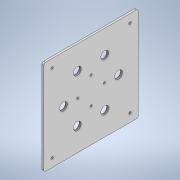
# Autodesk Inventor part: Plate
Saved by Autodesk Inventor 2022 (Build 260153000, 153)
## iProperties
Created: 2022-03-14
Part Number: Plate
Material: Generic
Document SubType Name: Modeling
Designer: ultra
Density: 1 g/cm^3
Appearance: Default
Author: ultra
Autodesk Inventor part; units mm, degrees
ref_plane "YZ Plane" through (0, 0, 0) normal (1, 0, 0) x (0, 1, 0)
ref_plane "XZ Plane" through (0, 0, 0) normal (0, 1, 0) x (-1, 0, 0)
ref_plane "XY Plane" through (0, 0, 0) normal (0, 0, 1) x (1, 0, 0)
sketch "Sketch1" plane through (0, 0, 0) normal (1, 0, 0) x (0, 1, 0)
  line L0 (-76.2, 76.2) -> (76.2, 76.2)
  line L1 (76.2, 76.2) -> (76.2, -76.2)
  line L2 (76.2, -76.2) -> (-76.2, -76.2)
  line L3 (-76.2, -76.2) -> (-76.2, 76.2)
  circle A0 centre (62.8611, 62.86) radius 2.032
  circle A1 centre (-62.8625, -62.8636) radius 2.032
  circle A2 centre (-0.0007, -88.9018) radius 2.032
  circle A3 centre (-62.8625, 62.86) radius 2.032
  circle A4 centre (88.8993, -0.0018) radius 2.032
  circle A5 centre (-88.9007, -0.0018) radius 2.032
  circle A6 centre (62.8611, -62.8636) radius 2.032
  circle A7 centre (-0.0007, 88.8982) radius 2.032
  circle A8 centre (-0.0007, -0.0018) radius 6.35
  dimension "d0" = 152.4
  dimension "d1" = 152.4
  dimension "d5" = 12.7
  constraints: 9 centre point, 8 end point, 2 parallel, 1 horizontal, 1 perpendicular
  measures "d0" distance of L1.end L2.end
  measures "d1" distance of L0.end L1.end
  measures "d5" diameter of A8
extrude "Extrusion2" add sketch "Sketch1" along normal blind 3.175 contours L0 L1 L2 L3 | A8
fillet "Fillet2" radius 3.175 4 edges at (1.5875, 76.2, 76.2) (1.5875, 76.2, -76.2) (1.5875, -76.2, 76.2) (1.5875, -76.2, -76.2)
sketch "Sketch2" plane through (3.175, 0, 0) normal (1, 0, 0) x (0, 0, -1)
  line L0 (-50.8, -50.8) -> (50.8, -50.8)
  line L1 (50.8, -50.8) -> (50.8, 50.8)
  line L2 (50.8, 50.8) -> (-50.8, 50.8)
  line L3 (-50.8, 50.8) -> (-50.8, -50.8)
  line L4 (-50.8, -50.8) -> (50.8, 50.8) construction
  line L5 (50.8, -50.8) -> (-50.8, 50.8) construction
  circle A0 centre (0, 0) radius 12.7
  line L6 (-12.7, 0) -> (-50.8, 38.1)
  line L7 (0, 12.7) -> (-38.1, 50.8)
  line L8 (-38.1, 50.8) -> (0, 12.7)
  line L9 (38.1, 50.8) -> (0, 12.7)
  line L10 (12.7, 0) -> (50.8, 38.1)
  line L11 (12.7, 0) -> (50.8, -38.1)
  line L12 (0, -12.7) -> (38.1, -50.8)
  line L13 (0, -12.7) -> (-38.1, -50.8)
  line L14 (-12.7, 0) -> (-50.8, -38.1)
  dimension "d9" = 101.6
  dimension "d10" = 101.6
  dimension "d11" = 25.4
  constraints: 30 end point, 10 point on line, 5 parallel, 4 point on circle, 2 midpoint, 2 perpendicular, 1 centre point, 1 coincident, 1 collinear, 1 horizontal
  measures "d9" distance of L2.end L1.end
  measures "d10" distance of L1.end L0.end
  measures "d11" diameter of A0
extrude "Extrusion3" [suppressed]
fillet "Fillet3" [suppressed]
sketch "Sketch3" plane through (3.175, 0, 0) normal (1, 0, 0) x (0, 0, -1)
  circle A0 centre (-22.225, -38.4948) radius 6.35
  circle A1 centre (-44.45, 0) radius 6.35
  circle A2 centre (22.225, -38.4948) radius 6.35
  circle A3 centre (-22.225, 38.4948) radius 6.35
  circle A4 centre (22.225, 38.4948) radius 6.35
  circle A5 centre (44.45, 0) radius 6.35
  point P0 (0, 0)
  constraints: 6 centre point
extrude "Extrusion4" cut sketch "Sketch3" against normal blind 25.4
sketch "Sketch4" plane through (3.175, 0, 0) normal (1, 0, 0) x (0, 0, -1)
  arc A0 (23.2155, 2.1696) -> (22.9916, -2.3228) centre (21.5668, 0) ccw
  line L0 (23.2155, 2.1696) -> (2.1696, 23.2155)
  arc A1 (-2.3228, 22.9916) -> (2.1696, 23.2155) centre (0, 21.5668) ccw
  line L1 (-2.3228, 22.9916) -> (-22.9916, 2.3228)
  arc A2 (-21.0224, -2.6701) -> (-22.9916, 2.3228) centre (-21.5668, 0) ccw
  arc A3 (-21.0026, -2.6855) -> (-21.0224, -2.6701) centre (-21.0733, -2.7562) ccw
  line L2 (-21.0026, -2.6855) -> (-2.6855, -21.0026)
  arc A4 (-2.6701, -21.0224) -> (-2.6855, -21.0026) centre (-2.7562, -21.0733) ccw
  arc A5 (2.3228, -22.9916) -> (-2.6701, -21.0224) centre (0, -21.5668) ccw
  line L3 (2.3228, -22.9916) -> (22.9916, -2.3228)
  circle A6 centre (3.0052, -18.703) radius 0.6
  circle A7 centre (4.1012, -19.799) radius 0.6
  circle A8 centre (6.8364, 2.2749) radius 0.5
  line L4 (-6.1377, 16.2493) -> (-7.0852, 17.1968)
  arc A9 (-6.1377, 16.1362) -> (-6.1377, 16.2493) centre (-6.1943, 16.1927) ccw
  line L5 (-7.0852, 15.1887) -> (-6.1377, 16.1362)
  arc A10 (-7.1983, 15.1887) -> (-7.0852, 15.1887) centre (-7.1418, 15.2452) ccw
  line L6 (-8.1459, 16.1362) -> (-7.1983, 15.1887)
  arc A11 (-8.1459, 16.2493) -> (-8.1459, 16.1362) centre (-8.0893, 16.1927) ccw
  line L7 (-7.1983, 17.1968) -> (-8.1459, 16.2493)
  arc A12 (-7.0852, 17.1968) -> (-7.1983, 17.1968) centre (-7.1418, 17.1403) ccw
  line L8 (8.8176, 15.6483) -> (7.8701, 16.5958)
  arc A13 (8.8176, 15.5351) -> (8.8176, 15.6483) centre (8.7611, 15.5917) ccw
  line L9 (7.8701, 14.5876) -> (8.8176, 15.5351)
  arc A14 (7.757, 14.5876) -> (7.8701, 14.5876) centre (7.8135, 14.6442) ccw
  line L10 (6.8094, 15.5351) -> (7.757, 14.5876)
  arc A15 (6.8094, 15.6483) -> (6.8094, 15.5351) centre (6.866, 15.5917) ccw
  line L11 (7.757, 16.5958) -> (6.8094, 15.6483)
  arc A16 (7.8701, 16.5958) -> (7.757, 16.5958) centre (7.8135, 16.5392) ccw
  line L12 (19.601, 4.7235) -> (18.6535, 5.671)
  arc A17 (19.601, 4.6103) -> (19.601, 4.7235) centre (19.5444, 4.6669) ccw
  line L13 (18.6535, 3.6628) -> (19.601, 4.6103)
  arc A18 (18.5403, 3.6628) -> (18.6535, 3.6628) centre (18.5969, 3.7194) ccw
  line L14 (17.5928, 4.6103) -> (18.5403, 3.6628)
  arc A19 (17.5928, 4.7235) -> (17.5928, 4.6103) centre (17.6494, 4.6669) ccw
  line L15 (18.5403, 5.671) -> (17.5928, 4.7235)
  arc A20 (18.6535, 5.671) -> (18.5403, 5.671) centre (18.5969, 5.6144) ccw
  line L16 (15.8533, 4.5821) -> (14.9058, 5.5296)
  arc A21 (15.8533, 4.4689) -> (15.8533, 4.5821) centre (15.7968, 4.5255) ccw
  line L17 (14.9058, 3.5214) -> (15.8533, 4.4689)
  arc A22 (14.7927, 3.5214) -> (14.9058, 3.5214) centre (14.8492, 3.578) ccw
  line L18 (13.8452, 4.4689) -> (14.7927, 3.5214)
  arc A23 (13.8452, 4.5821) -> (13.8452, 4.4689) centre (13.9017, 4.5255) ccw
  line L19 (14.7927, 5.5296) -> (13.8452, 4.5821)
  arc A24 (14.9058, 5.5296) -> (14.7927, 5.5296) centre (14.8492, 5.473) ccw
  line L20 (16.419, 0.1273) -> (15.4715, 1.0748)
  arc A25 (16.419, 0.0141) -> (16.419, 0.1273) centre (16.3625, 0.0707) ccw
  line L21 (15.4715, -0.9334) -> (16.419, 0.0141)
  arc A26 (15.3584, -0.9334) -> (15.4715, -0.9334) centre (15.4149, -0.8768) ccw
  line L22 (14.4108, 0.0141) -> (15.3584, -0.9334)
  arc A27 (14.4108, 0.1273) -> (14.4108, 0.0141) centre (14.4674, 0.0707) ccw
  line L23 (15.3584, 1.0748) -> (14.4108, 0.1273)
  arc A28 (15.4715, 1.0748) -> (15.3584, 1.0748) centre (15.4149, 1.0182) ccw
  circle A29 centre (16.122, -7.2832) radius 0.75
  circle A30 centre (-6.5407, -11.7733) radius 0.6
  circle A31 centre (-7.6014, -10.7127) radius 0.6
  circle A32 centre (-8.6621, -9.652) radius 0.6
  circle A33 centre (-8.8035, -12.4097) radius 0.5
  line L24 (18.9292, -5.4235) -> (17.9817, -4.476)
  arc A34 (18.9292, -5.5366) -> (18.9292, -5.4235) centre (18.8727, -5.4801) ccw
  line L25 (17.9817, -6.4842) -> (18.9292, -5.5366)
  arc A35 (17.8686, -6.4842) -> (17.9817, -6.4842) centre (17.9252, -6.4276) ccw
  line L26 (16.9211, -5.5366) -> (17.8686, -6.4842)
  arc A36 (16.9211, -5.4235) -> (16.9211, -5.5366) centre (16.9776, -5.4801) ccw
  line L27 (17.8686, -4.476) -> (16.9211, -5.4235)
  arc A37 (17.9817, -4.476) -> (17.8686, -4.476) centre (17.9252, -4.5326) ccw
  line L28 (-4.2144, 14.326) -> (-5.1619, 15.2735)
  arc A38 (-4.2144, 14.2128) -> (-4.2144, 14.326) centre (-4.2709, 14.2694) ccw
  line L29 (-5.1619, 13.2653) -> (-4.2144, 14.2128)
  arc A39 (-5.275, 13.2653) -> (-5.1619, 13.2653) centre (-5.2184, 13.3219) ccw
  line L30 (-6.2225, 14.2128) -> (-5.275, 13.2653)
  arc A40 (-6.2225, 14.326) -> (-6.2225, 14.2128) centre (-6.166, 14.2694) ccw
  line L31 (-5.275, 15.2735) -> (-6.2225, 14.326)
  arc A41 (-5.1619, 15.2735) -> (-5.275, 15.2735) centre (-5.2184, 15.2169) ccw
  line L32 (7.3618, 0.623) -> (8.3055, 1.5667)
  arc A42 (7.2487, 0.623) -> (7.3618, 0.623) centre (7.3053, 0.6795) ccw
  line L33 (6.8654, 1.0063) -> (7.2487, 0.623)
  arc A43 (6.8654, 1.1194) -> (6.8654, 1.0063) centre (6.922, 1.0629) ccw
  line L34 (7.8091, 2.0631) -> (6.8654, 1.1194)
  arc A44 (7.9222, 2.0631) -> (7.8091, 2.0631) centre (7.8657, 2.0066) ccw
  line L35 (8.3055, 1.6798) -> (7.9222, 2.0631)
  arc A45 (8.3055, 1.5667) -> (8.3055, 1.6798) centre (8.249, 1.6232) ccw
  line L36 (12.9068, -4.7667) -> (14.116, -3.5576)
  arc A46 (12.7937, -4.7667) -> (12.9068, -4.7667) centre (12.8503, -4.7101) ccw
  line L37 (12.0957, -4.0687) -> (12.7937, -4.7667)
  arc A47 (12.0957, -3.9555) -> (12.0957, -4.0687) centre (12.1522, -4.0121) ccw
  line L38 (13.3048, -2.7464) -> (12.0957, -3.9555)
  arc A48 (13.4179, -2.7464) -> (13.3048, -2.7464) centre (13.3614, -2.803) ccw
  line L39 (14.116, -3.4444) -> (13.4179, -2.7464)
  arc A49 (14.116, -3.5576) -> (14.116, -3.4444) centre (14.0594, -3.501) ccw
  line L40 (6.6373, -11.9558) -> (4.8803, -13.7127)
  arc A50 (6.8494, -11.9558) -> (6.6373, -11.9558) centre (6.7433, -12.0618) ccw
  line L41 (7.3, -12.4064) -> (6.8494, -11.9558)
  arc A51 (7.3, -12.6185) -> (7.3, -12.4064) centre (7.194, -12.5125) ccw
  line L42 (5.5431, -14.3755) -> (7.3, -12.6185)
  arc A52 (5.3309, -14.3755) -> (5.5431, -14.3755) centre (5.437, -14.2694) ccw
  line L43 (4.8803, -13.9248) -> (5.3309, -14.3755)
  arc A53 (4.8803, -13.7127) -> (4.8803, -13.9248) centre (4.9864, -13.8188) ccw
  line L44 (-10.9165, -1.3583) -> (-10.3201, -0.7619)
  arc A54 (-11.0296, -1.3583) -> (-10.9165, -1.3583) centre (-10.973, -1.3017) ccw
  line L45 (-11.2566, -1.1313) -> (-11.0296, -1.3583)
  arc A55 (-11.2566, -1.0181) -> (-11.2566, -1.1313) centre (-11.2001, -1.0747) ccw
  line L46 (-10.6602, -0.4217) -> (-11.2566, -1.0181)
  arc A56 (-10.5471, -0.4217) -> (-10.6602, -0.4217) centre (-10.6037, -0.4783) ccw
  line L47 (-10.3201, -0.6487) -> (-10.5471, -0.4217)
  arc A57 (-10.3201, -0.7619) -> (-10.3201, -0.6487) centre (-10.3766, -0.7053) ccw
  line L48 (-10.4537, -1.8887) -> (-10.2266, -2.1157)
  arc A58 (-10.4537, -1.7755) -> (-10.4537, -1.8887) centre (-10.3971, -1.8321) ccw
  line L49 (-9.8573, -1.1791) -> (-10.4537, -1.7755)
  arc A59 (-9.7441, -1.1791) -> (-9.8573, -1.1791) centre (-9.8007, -1.2357) ccw
  line L50 (-9.5171, -1.4061) -> (-9.7441, -1.1791)
  arc A60 (-9.5171, -1.5193) -> (-9.5171, -1.4061) centre (-9.5737, -1.4627) ccw
  line L51 (-10.1135, -2.1157) -> (-9.5171, -1.5193)
  arc A61 (-10.2266, -2.1157) -> (-10.1135, -2.1157) centre (-10.1701, -2.0591) ccw
  line L52 (-4.4405, 1.0113) -> (-4.2546, 0.8254)
  arc A62 (-4.4405, 1.1244) -> (-4.4405, 1.0113) centre (-4.384, 1.0679) ccw
  line L53 (-3.9397, 1.6252) -> (-4.4405, 1.1244)
  arc A63 (-3.8266, 1.6252) -> (-3.9397, 1.6252) centre (-3.8832, 1.5686) ccw
  line L54 (-3.6407, 1.4393) -> (-3.8266, 1.6252)
  arc A64 (-3.6407, 1.3261) -> (-3.6407, 1.4393) centre (-3.6972, 1.3827) ccw
  line L55 (-4.1415, 0.8254) -> (-3.6407, 1.3261)
  arc A65 (-4.2546, 0.8254) -> (-4.1415, 0.8254) centre (-4.198, 0.8819) ccw
  line L56 (-8.9918, 6.0077) -> (-8.8058, 5.8218)
  arc A66 (-8.9918, 6.1208) -> (-8.9918, 6.0077) centre (-8.9352, 6.0642) ccw
  line L57 (-8.491, 6.6216) -> (-8.9918, 6.1208)
  arc A67 (-8.3778, 6.6216) -> (-8.491, 6.6216) centre (-8.4344, 6.565) ccw
  line L58 (-8.1919, 6.4357) -> (-8.3778, 6.6216)
  arc A68 (-8.1919, 6.3225) -> (-8.1919, 6.4357) centre (-8.2485, 6.3791) ccw
  line L59 (-8.6927, 5.8218) -> (-8.1919, 6.3225)
  arc A69 (-8.8058, 5.8218) -> (-8.6927, 5.8218) centre (-8.7493, 5.8783) ccw
  line L60 (2.8669, 3.1449) -> (3.0528, 2.9589)
  arc A70 (2.8669, 3.258) -> (2.8669, 3.1449) centre (2.9235, 3.2014) ccw
  line L61 (3.3677, 3.7588) -> (2.8669, 3.258)
  arc A71 (3.4808, 3.7588) -> (3.3677, 3.7588) centre (3.4243, 3.7022) ccw
  line L62 (3.6668, 3.5729) -> (3.4808, 3.7588)
  arc A72 (3.6668, 3.4597) -> (3.6668, 3.5729) centre (3.6102, 3.5163) ccw
  line L63 (3.166, 2.9589) -> (3.6668, 3.4597)
  arc A73 (3.0528, 2.9589) -> (3.166, 2.9589) centre (3.1094, 3.0155) ccw
  line L64 (4.4253, 1.5865) -> (4.6112, 1.4005)
  arc A74 (4.4253, 1.6996) -> (4.4253, 1.5865) centre (4.4819, 1.643) ccw
  line L65 (4.9261, 2.2004) -> (4.4253, 1.6996)
  arc A75 (5.0392, 2.2004) -> (4.9261, 2.2004) centre (4.9827, 2.1438) ccw
  line L66 (5.2252, 2.0145) -> (5.0392, 2.2004)
  arc A76 (5.2252, 1.9013) -> (5.2252, 2.0145) centre (5.1686, 1.9579) ccw
  line L67 (4.7244, 1.4005) -> (5.2252, 1.9013)
  arc A77 (4.6112, 1.4005) -> (4.7244, 1.4005) centre (4.6678, 1.4571) ccw
  line L68 (7.7498, 0.1218) -> (7.9358, -0.0641)
  arc A78 (7.7498, 0.235) -> (7.7498, 0.1218) centre (7.8064, 0.1784) ccw
  line L69 (8.2506, 0.7358) -> (7.7498, 0.235)
  arc A79 (8.3638, 0.7358) -> (8.2506, 0.7358) centre (8.3072, 0.6792) ccw
  line L70 (8.5497, 0.5498) -> (8.3638, 0.7358)
  arc A80 (8.5497, 0.4367) -> (8.5497, 0.5498) centre (8.4931, 0.4933) ccw
  line L71 (8.0489, -0.0641) -> (8.5497, 0.4367)
  arc A81 (7.9358, -0.0641) -> (8.0489, -0.0641) centre (7.9923, -0.0075) ccw
  line L72 (11.3694, -3.4478) -> (11.5553, -3.6337)
  arc A82 (11.3694, -3.3347) -> (11.3694, -3.4478) centre (11.426, -3.3912) ccw
  line L73 (11.8702, -2.8339) -> (11.3694, -3.3347)
  arc A83 (11.9833, -2.8339) -> (11.8702, -2.8339) centre (11.9268, -2.8904) ccw
  line L74 (12.1692, -3.0198) -> (11.9833, -2.8339)
  arc A84 (12.1692, -3.1329) -> (12.1692, -3.0198) centre (12.1127, -3.0764) ccw
  line L75 (11.6685, -3.6337) -> (12.1692, -3.1329)
  arc A85 (11.5553, -3.6337) -> (11.6685, -3.6337) centre (11.6119, -3.5771) ccw
  line L76 (7.2531, -10.8075) -> (7.439, -10.9935)
  arc A86 (7.2531, -10.6944) -> (7.2531, -10.8075) centre (7.3097, -10.751) ccw
  line L77 (7.7539, -10.1936) -> (7.2531, -10.6944)
  arc A87 (7.867, -10.1936) -> (7.7539, -10.1936) centre (7.8105, -10.2502) ccw
  line L78 (8.053, -10.3795) -> (7.867, -10.1936)
  arc A88 (8.053, -10.4927) -> (8.053, -10.3795) centre (7.9964, -10.4361) ccw
  line L79 (7.5522, -10.9935) -> (8.053, -10.4927)
  arc A89 (7.439, -10.9935) -> (7.5522, -10.9935) centre (7.4956, -10.9369) ccw
  line L80 (8.0117, -11.5935) -> (8.2265, -11.8083)
  arc A90 (8.0117, -11.4804) -> (8.0117, -11.5935) centre (8.0683, -11.537) ccw
  line L81 (8.5536, -10.9385) -> (8.0117, -11.4804)
  arc A91 (8.6668, -10.9385) -> (8.5536, -10.9385) centre (8.6102, -10.995) ccw
  line L82 (8.8816, -11.1533) -> (8.6668, -10.9385)
  arc A92 (8.8816, -11.2664) -> (8.8816, -11.1533) centre (8.825, -11.2098) ccw
  line L83 (8.3396, -11.8083) -> (8.8816, -11.2664)
  arc A93 (8.2265, -11.8083) -> (8.3396, -11.8083) centre (8.2831, -11.7518) ccw
  line L84 (-8.0565, 2.0509) -> (-7.8655, 2.2419)
  arc A94 (-8.1696, 2.0509) -> (-8.0565, 2.0509) centre (-8.1131, 2.1075) ccw
  line L85 (-8.6663, 2.5475) -> (-8.1696, 2.0509)
  arc A95 (-8.6663, 2.6607) -> (-8.6663, 2.5475) centre (-8.6097, 2.6041) ccw
  line L86 (-8.4753, 2.8517) -> (-8.6663, 2.6607)
  arc A96 (-8.3622, 2.8517) -> (-8.4753, 2.8517) centre (-8.4187, 2.7951) ccw
  line L87 (-7.8655, 2.355) -> (-8.3622, 2.8517)
  arc A97 (-7.8655, 2.2419) -> (-7.8655, 2.355) centre (-7.9221, 2.2985) ccw
  line L88 (-6.485, 0.2962) -> (-5.9884, -0.2005)
  arc A98 (-6.485, 0.4093) -> (-6.485, 0.2962) centre (-6.4285, 0.3527) ccw
  line L89 (-6.294, 0.6003) -> (-6.485, 0.4093)
  arc A99 (-6.1809, 0.6003) -> (-6.294, 0.6003) centre (-6.2375, 0.5437) ccw
  line L90 (-5.6842, 0.1036) -> (-6.1809, 0.6003)
  arc A100 (-5.6842, -0.0095) -> (-5.6842, 0.1036) centre (-5.7408, 0.0471) ccw
  line L91 (-5.8752, -0.2005) -> (-5.6842, -0.0095)
  arc A101 (-5.9884, -0.2005) -> (-5.8752, -0.2005) centre (-5.9318, -0.1439) ccw
  line L92 (-8.0538, -3.0609) -> (-7.5571, -3.5576)
  arc A102 (-8.0538, -2.9478) -> (-8.0538, -3.0609) centre (-7.9972, -3.0044) ccw
  line L93 (-7.8627, -2.7568) -> (-8.0538, -2.9478)
  arc A103 (-7.7496, -2.7568) -> (-7.8627, -2.7568) centre (-7.8062, -2.8133) ccw
  line L94 (-7.253, -3.2534) -> (-7.7496, -2.7568)
  arc A104 (-7.253, -3.3666) -> (-7.253, -3.2534) centre (-7.3095, -3.31) ccw
  line L95 (-7.444, -3.5576) -> (-7.253, -3.3666)
  arc A105 (-7.5571, -3.5576) -> (-7.444, -3.5576) centre (-7.5005, -3.501) ccw
  line L96 (10.6894, 0.9692) -> (11.186, 0.4725)
  arc A106 (10.6894, 1.0823) -> (10.6894, 0.9692) centre (10.746, 1.0257) ccw
  line L97 (10.8804, 1.2733) -> (10.6894, 1.0823)
  arc A107 (10.9935, 1.2733) -> (10.8804, 1.2733) centre (10.937, 1.2167) ccw
  line L98 (11.4902, 0.7766) -> (10.9935, 1.2733)
  arc A108 (11.4902, 0.6635) -> (11.4902, 0.7766) centre (11.4336, 0.7201) ccw
  line L99 (11.2992, 0.4725) -> (11.4902, 0.6635)
  arc A109 (11.186, 0.4725) -> (11.2992, 0.4725) centre (11.2426, 0.5291) ccw
  line L100 (7.9785, -2.1827) -> (8.4752, -2.6794)
  arc A110 (7.9785, -2.0696) -> (7.9785, -2.1827) centre (8.0351, -2.1261) ccw
  line L101 (8.1696, -1.8785) -> (7.9785, -2.0696)
  arc A111 (8.2827, -1.8785) -> (8.1696, -1.8785) centre (8.2261, -1.9351) ccw
  line L102 (8.7793, -2.3752) -> (8.2827, -1.8785)
  arc A112 (8.7793, -2.4883) -> (8.7793, -2.3752) centre (8.7228, -2.4318) ccw
  line L103 (8.5883, -2.6794) -> (8.7793, -2.4883)
  arc A113 (8.4752, -2.6794) -> (8.5883, -2.6794) centre (8.5318, -2.6228) ccw
  line L104 (10.502, -8.0563) -> (10.9987, -8.5529)
  arc A114 (10.502, -7.9431) -> (10.502, -8.0563) centre (10.5586, -7.9997) ccw
  line L105 (10.693, -7.7521) -> (10.502, -7.9431)
  arc A115 (10.8061, -7.7521) -> (10.693, -7.7521) centre (10.7496, -7.8087) ccw
  line L106 (11.3028, -8.2488) -> (10.8061, -7.7521)
  arc A116 (11.3028, -8.3619) -> (11.3028, -8.2488) centre (11.2462, -8.3054) ccw
  line L107 (11.1118, -8.5529) -> (11.3028, -8.3619)
  arc A117 (10.9987, -8.5529) -> (11.1118, -8.5529) centre (11.0552, -8.4964) ccw
  line L108 (9.7298, -8.8285) -> (10.2265, -9.3251)
  arc A118 (9.7298, -8.7153) -> (9.7298, -8.8285) centre (9.7864, -8.7719) ccw
  line L109 (9.9208, -8.5243) -> (9.7298, -8.7153)
  arc A119 (10.034, -8.5243) -> (9.9208, -8.5243) centre (9.9774, -8.5809) ccw
  line L110 (10.5306, -9.021) -> (10.034, -8.5243)
  arc A120 (10.5306, -9.1341) -> (10.5306, -9.021) centre (10.474, -9.0776) ccw
  line L111 (10.3396, -9.3251) -> (10.5306, -9.1341)
  arc A121 (10.2265, -9.3251) -> (10.3396, -9.3251) centre (10.283, -9.2686) ccw
  line L112 (8.8271, -9.6036) -> (9.4328, -10.2093)
  arc A122 (8.8271, -9.4905) -> (8.8271, -9.6036) centre (8.8837, -9.5471) ccw
  line L113 (9.1377, -9.1799) -> (8.8271, -9.4905)
  arc A123 (9.2508, -9.1799) -> (9.1377, -9.1799) centre (9.1943, -9.2365) ccw
  line L114 (9.8566, -9.7856) -> (9.2508, -9.1799)
  arc A124 (9.8566, -9.8987) -> (9.8566, -9.7856) centre (9.8, -9.8422) ccw
  line L115 (9.5459, -10.2093) -> (9.8566, -9.8987)
  arc A125 (9.4328, -10.2093) -> (9.5459, -10.2093) centre (9.4894, -10.1528) ccw
  line L116 (3.8806, -14.6777) -> (4.3772, -15.1744)
  arc A126 (3.8806, -14.5646) -> (3.8806, -14.6777) centre (3.9371, -14.6211) ccw
  line L117 (4.0716, -14.3736) -> (3.8806, -14.5646)
  arc A127 (4.1847, -14.3736) -> (4.0716, -14.3736) centre (4.1281, -14.4301) ccw
  line L118 (4.6814, -14.8702) -> (4.1847, -14.3736)
  arc A128 (4.6814, -14.9834) -> (4.6814, -14.8702) centre (4.6248, -14.9268) ccw
  line L119 (4.4904, -15.1744) -> (4.6814, -14.9834)
  arc A129 (4.3772, -15.1744) -> (4.4904, -15.1744) centre (4.4338, -15.1178) ccw
  line L120 (-2.5721, -13.7107) -> (-2.0754, -14.2074)
  arc A130 (-2.5721, -13.5976) -> (-2.5721, -13.7107) centre (-2.5155, -13.6542) ccw
  line L121 (-2.3811, -13.4066) -> (-2.5721, -13.5976)
  arc A131 (-2.2679, -13.4066) -> (-2.3811, -13.4066) centre (-2.3245, -13.4631) ccw
  line L122 (-1.7713, -13.9032) -> (-2.2679, -13.4066)
  arc A132 (-1.7713, -14.0164) -> (-1.7713, -13.9032) centre (-1.8279, -13.9598) ccw
  line L123 (-1.9623, -14.2074) -> (-1.7713, -14.0164)
  arc A133 (-2.0754, -14.2074) -> (-1.9623, -14.2074) centre (-2.0189, -14.1508) ccw
  line L124 (-4.0504, -12.2324) -> (-3.5538, -12.729)
  arc A134 (-4.0504, -12.1192) -> (-4.0504, -12.2324) centre (-3.9939, -12.1758) ccw
  line L125 (-3.8594, -11.9282) -> (-4.0504, -12.1192)
  arc A135 (-3.7463, -11.9282) -> (-3.8594, -11.9282) centre (-3.8029, -11.9848) ccw
  line L126 (-3.2496, -12.4249) -> (-3.7463, -11.9282)
  arc A136 (-3.2496, -12.538) -> (-3.2496, -12.4249) centre (-3.3062, -12.4815) ccw
  line L127 (-3.4406, -12.729) -> (-3.2496, -12.538)
  arc A137 (-3.5538, -12.729) -> (-3.4406, -12.729) centre (-3.4972, -12.6725) ccw
  line L128 (-6.708, -2.9151) -> (-6.4115, -2.6186)
  arc A138 (-6.8211, -2.9151) -> (-6.708, -2.9151) centre (-6.7645, -2.8585) ccw
  line L129 (-7.4165, -2.3197) -> (-6.8211, -2.9151)
  arc A139 (-7.4165, -2.2066) -> (-7.4165, -2.3197) centre (-7.3599, -2.2631) ccw
  line L130 (-7.12, -1.9101) -> (-7.4165, -2.2066)
  arc A140 (-7.0069, -1.9101) -> (-7.12, -1.9101) centre (-7.0634, -1.9667) ccw
  line L131 (-6.4115, -2.5055) -> (-7.0069, -1.9101)
  arc A141 (-6.4115, -2.6186) -> (-6.4115, -2.5055) centre (-6.468, -2.5621) ccw
  line L132 (3.9359, 2.0688) -> (4.5587, 2.6916)
  arc A142 (3.8227, 2.0688) -> (3.9359, 2.0688) centre (3.8793, 2.1253) ccw
  line L133 (3.5244, 2.3671) -> (3.8227, 2.0688)
  arc A143 (3.5244, 2.4802) -> (3.5244, 2.3671) centre (3.5809, 2.4237) ccw
  line L134 (4.1472, 3.1031) -> (3.5244, 2.4802)
  arc A144 (4.2603, 3.1031) -> (4.1472, 3.1031) centre (4.2038, 3.0465) ccw
  line L135 (4.5587, 2.8047) -> (4.2603, 3.1031)
  arc A145 (4.5587, 2.6916) -> (4.5587, 2.8047) centre (4.5021, 2.7482) ccw
  line L136 (-2.7105, 14.8239) -> (-2.1795, 15.3549)
  arc A146 (-2.8236, 14.8239) -> (-2.7105, 14.8239) centre (-2.767, 14.8805) ccw
  line L137 (-3.7755, 15.7758) -> (-2.8236, 14.8239)
  arc A147 (-3.7755, 15.8889) -> (-3.7755, 15.7758) centre (-3.7189, 15.8324) ccw
  line L138 (-3.2445, 16.4199) -> (-3.7755, 15.8889)
  arc A148 (-3.1314, 16.4199) -> (-3.2445, 16.4199) centre (-3.1879, 16.3633) ccw
  line L139 (-2.1795, 15.468) -> (-3.1314, 16.4199)
  arc A149 (-2.1795, 15.3549) -> (-2.1795, 15.468) centre (-2.2361, 15.4115) ccw
  line L140 (-4.6244, 16.7379) -> (-4.1517, 17.2106)
  arc A150 (-4.7376, 16.7379) -> (-4.6244, 16.7379) centre (-4.681, 16.7945) ccw
  line L141 (-5.7487, 17.749) -> (-4.7376, 16.7379)
  arc A151 (-5.7487, 17.8621) -> (-5.7487, 17.749) centre (-5.6921, 17.8056) ccw
  line L142 (-5.276, 18.3349) -> (-5.7487, 17.8621)
  arc A152 (-5.1628, 18.3349) -> (-5.276, 18.3349) centre (-5.2194, 18.2783) ccw
  line L143 (-4.1517, 17.3237) -> (-5.1628, 18.3349)
  arc A153 (-4.1517, 17.2106) -> (-4.1517, 17.3237) centre (-4.2083, 17.2672) ccw
  line L144 (-4.9285, 9.382) -> (-4.7198, 9.5906)
  arc A154 (-5.0416, 9.382) -> (-4.9285, 9.382) centre (-4.985, 9.4386) ccw
  line L145 (-5.5864, 9.9267) -> (-5.0416, 9.382)
  arc A155 (-5.5864, 10.0399) -> (-5.5864, 9.9267) centre (-5.5298, 9.9833) ccw
  line L146 (-5.3777, 10.2485) -> (-5.5864, 10.0399)
  arc A156 (-5.2646, 10.2485) -> (-5.3777, 10.2485) centre (-5.3212, 10.1919) ccw
  line L147 (-4.7198, 9.7038) -> (-5.2646, 10.2485)
  arc A157 (-4.7198, 9.5906) -> (-4.7198, 9.7038) centre (-4.7764, 9.6472) ccw
  line L148 (-4.7907, 10.6822) -> (-4.246, 10.1374)
  arc A158 (-4.7907, 10.7953) -> (-4.7907, 10.6822) centre (-4.7341, 10.7387) ccw
  line L149 (-4.5821, 11.0039) -> (-4.7907, 10.7953)
  arc A159 (-4.4689, 11.0039) -> (-4.5821, 11.0039) centre (-4.5255, 10.9474) ccw
  line L150 (-3.9242, 10.4592) -> (-4.4689, 11.0039)
  arc A160 (-3.9242, 10.3461) -> (-3.9242, 10.4592) centre (-3.9808, 10.4026) ccw
  line L151 (-4.1328, 10.1374) -> (-3.9242, 10.3461)
  arc A161 (-4.246, 10.1374) -> (-4.1328, 10.1374) centre (-4.1894, 10.194) ccw
  line L152 (-4.0149, 11.458) -> (-3.4701, 10.9132)
  arc A162 (-4.0149, 11.5711) -> (-4.0149, 11.458) centre (-3.9583, 11.5146) ccw
  line L153 (-3.8063, 11.7797) -> (-4.0149, 11.5711)
  arc A163 (-3.6931, 11.7797) -> (-3.8063, 11.7797) centre (-3.7497, 11.7232) ccw
  line L154 (-3.1484, 11.235) -> (-3.6931, 11.7797)
  arc A164 (-3.1484, 11.1219) -> (-3.1484, 11.235) centre (-3.205, 11.1784) ccw
  line L155 (-3.357, 10.9132) -> (-3.1484, 11.1219)
  arc A165 (-3.4701, 10.9132) -> (-3.357, 10.9132) centre (-3.4136, 10.9698) ccw
  line L156 (-2.9863, 12.4866) -> (-2.4416, 11.9418)
  arc A166 (-2.9863, 12.5997) -> (-2.9863, 12.4866) centre (-2.9297, 12.5431) ccw
  line L157 (-2.7777, 12.8083) -> (-2.9863, 12.5997)
  arc A167 (-2.6646, 12.8083) -> (-2.7777, 12.8083) centre (-2.7211, 12.7518) ccw
  line L158 (-2.1198, 12.2636) -> (-2.6646, 12.8083)
  arc A168 (-2.1198, 12.1504) -> (-2.1198, 12.2636) centre (-2.1764, 12.207) ccw
  line L159 (-2.3284, 11.9418) -> (-2.1198, 12.1504)
  arc A169 (-2.4416, 11.9418) -> (-2.3284, 11.9418) centre (-2.385, 11.9984) ccw
  line L160 (-2.2113, 13.1966) -> (-1.6665, 12.6519)
  arc A170 (-2.2113, 13.3098) -> (-2.2113, 13.1966) centre (-2.1547, 13.2532) ccw
  line L161 (-2.0026, 13.5184) -> (-2.2113, 13.3098)
  arc A171 (-1.8895, 13.5184) -> (-2.0026, 13.5184) centre (-1.9461, 13.4618) ccw
  line L162 (-1.3447, 12.9736) -> (-1.8895, 13.5184)
  arc A172 (-1.3447, 12.8605) -> (-1.3447, 12.9736) centre (-1.4013, 12.9171) ccw
  line L163 (-1.5534, 12.6519) -> (-1.3447, 12.8605)
  arc A173 (-1.6665, 12.6519) -> (-1.5534, 12.6519) centre (-1.6099, 12.7084) ccw
  line L164 (-3.2047, 9.0962) -> (-2.66, 8.5514)
  arc A174 (-3.2047, 9.2093) -> (-3.2047, 9.0962) centre (-3.1482, 9.1528) ccw
  line L165 (-2.9961, 9.418) -> (-3.2047, 9.2093)
  arc A175 (-2.883, 9.418) -> (-2.9961, 9.418) centre (-2.9395, 9.3614) ccw
  line L166 (-2.3382, 8.8732) -> (-2.883, 9.418)
  arc A176 (-2.3382, 8.7601) -> (-2.3382, 8.8732) centre (-2.3948, 8.8166) ccw
  line L167 (-2.5468, 8.5514) -> (-2.3382, 8.7601)
  arc A177 (-2.66, 8.5514) -> (-2.5468, 8.5514) centre (-2.6034, 8.608) ccw
  line L168 (-1.7542, 7.6122) -> (-1.2095, 7.0674)
  arc A178 (-1.7542, 7.7253) -> (-1.7542, 7.6122) centre (-1.6977, 7.6688) ccw
  line L169 (-1.5456, 7.9339) -> (-1.7542, 7.7253)
  arc A179 (-1.4325, 7.9339) -> (-1.5456, 7.9339) centre (-1.4891, 7.8774) ccw
  line L170 (-0.8877, 7.3892) -> (-1.4325, 7.9339)
  arc A180 (-0.8877, 7.2761) -> (-0.8877, 7.3892) centre (-0.9443, 7.3326) ccw
  line L171 (-1.0964, 7.0674) -> (-0.8877, 7.2761)
  arc A181 (-1.2095, 7.0674) -> (-1.0964, 7.0674) centre (-1.1529, 7.124) ccw
  line L172 (13.279, -7.1541) -> (14.2033, -6.2298)
  arc A182 (13.1659, -7.1541) -> (13.279, -7.1541) centre (13.2224, -7.0975) ccw
  line L173 (12.7221, -6.7104) -> (13.1659, -7.1541)
  arc A183 (12.7221, -6.5972) -> (12.7221, -6.7104) centre (12.7787, -6.6538) ccw
  line L174 (13.6464, -5.6729) -> (12.7221, -6.5972)
  arc A184 (13.7595, -5.6729) -> (13.6464, -5.6729) centre (13.703, -5.7295) ccw
  line L175 (14.2033, -6.1167) -> (13.7595, -5.6729)
  arc A185 (14.2033, -6.2298) -> (14.2033, -6.1167) centre (14.1467, -6.1732) ccw
  line L176 (15.2014, -5.2317) -> (16.2064, -4.2266)
  arc A186 (15.0883, -5.2317) -> (15.2014, -5.2317) centre (15.1448, -5.1751) ccw
  line L177 (14.6446, -4.7879) -> (15.0883, -5.2317)
  arc A187 (14.6446, -4.6748) -> (14.6446, -4.7879) centre (14.7011, -4.7314) ccw
  line L178 (15.6496, -3.6698) -> (14.6446, -4.6748)
  arc A188 (15.7627, -3.6698) -> (15.6496, -3.6698) centre (15.7061, -3.7264) ccw
  line L179 (16.2064, -4.1135) -> (15.7627, -3.6698)
  arc A189 (16.2064, -4.2266) -> (16.2064, -4.1135) centre (16.1499, -4.1701) ccw
  line L180 (9.2038, 13.4854) -> (8.8721, 13.8171)
  line L181 (9.7139, 13.9956) -> (9.2038, 13.4854)
  arc A190 (9.9603, 13.9956) -> (9.7139, 13.9956) centre (9.8371, 13.8724) ccw
  line L182 (10.0834, 13.8724) -> (9.9603, 13.9956)
  arc A191 (10.0834, 13.6261) -> (10.0834, 13.8724) centre (9.9603, 13.7492) ccw
  line L183 (9.5733, 13.1159) -> (10.0834, 13.6261)
  line L184 (10.1035, 12.5857) -> (9.5733, 13.1159)
  line L185 (10.6137, 13.0958) -> (10.1035, 12.5857)
  arc A192 (10.86, 13.0958) -> (10.6137, 13.0958) centre (10.7368, 12.9727) ccw
  line L186 (10.9831, 12.9727) -> (10.86, 13.0958)
  arc A193 (10.9831, 12.7263) -> (10.9831, 12.9727) centre (10.86, 12.8495) ccw
  line L187 (10.473, 12.2162) -> (10.9831, 12.7263)
  line L188 (11.0032, 11.686) -> (10.473, 12.2162)
  line L189 (11.5134, 12.1961) -> (11.0032, 11.686)
  arc A194 (11.7597, 12.1961) -> (11.5134, 12.1961) centre (11.6365, 12.0729) ccw
  line L190 (11.8829, 12.0729) -> (11.7597, 12.1961)
  arc A195 (11.8829, 11.8266) -> (11.8829, 12.0729) centre (11.7597, 11.9498) ccw
  line L191 (11.3727, 11.3165) -> (11.8829, 11.8266)
  line L192 (11.903, 10.7862) -> (11.3727, 11.3165)
  line L193 (12.4131, 11.2964) -> (11.903, 10.7862)
  arc A196 (12.6594, 11.2964) -> (12.4131, 11.2964) centre (12.5363, 11.1732) ccw
  line L194 (12.7826, 11.1732) -> (12.6594, 11.2964)
  arc A197 (12.7826, 10.9269) -> (12.7826, 11.1732) centre (12.6594, 11.05) ccw
  line L195 (12.2725, 10.4167) -> (12.7826, 10.9269)
  line L196 (12.8027, 9.8865) -> (12.2725, 10.4167)
  line L197 (13.3128, 10.3966) -> (12.8027, 9.8865)
  arc A198 (13.5592, 10.3966) -> (13.3128, 10.3966) centre (13.436, 10.2735) ccw
  line L198 (13.6823, 10.2735) -> (13.5592, 10.3966)
  arc A199 (13.6823, 10.0272) -> (13.6823, 10.2735) centre (13.5592, 10.1503) ccw
  line L199 (13.1722, 9.517) -> (13.6823, 10.0272)
  line L200 (13.6598, 9.0294) -> (13.1722, 9.517)
  line L201 (11.5403, 6.9099) -> (13.6598, 9.0294)
  line L202 (11.0527, 7.3976) -> (11.5403, 6.9099)
  line L203 (10.5426, 6.8874) -> (11.0527, 7.3976)
  arc A200 (10.2963, 6.8874) -> (10.5426, 6.8874) centre (10.4194, 7.0106) ccw
  line L204 (10.1731, 7.0106) -> (10.2963, 6.8874)
  arc A201 (10.1731, 7.2569) -> (10.1731, 7.0106) centre (10.2963, 7.1337) ccw
  line L205 (10.6832, 7.767) -> (10.1731, 7.2569)
  line L206 (10.153, 8.2973) -> (10.6832, 7.767)
  line L207 (9.6429, 7.7871) -> (10.153, 8.2973)
  arc A202 (9.3965, 7.7871) -> (9.6429, 7.7871) centre (9.5197, 7.9103) ccw
  line L208 (9.2734, 7.9103) -> (9.3965, 7.7871)
  arc A203 (9.2734, 8.1566) -> (9.2734, 7.9103) centre (9.3965, 8.0335) ccw
  line L209 (9.7835, 8.6668) -> (9.2734, 8.1566)
  line L210 (9.2533, 9.197) -> (9.7835, 8.6668)
  line L211 (8.7431, 8.6869) -> (9.2533, 9.197)
  arc A204 (8.4968, 8.6869) -> (8.7431, 8.6869) centre (8.62, 8.81) ccw
  line L212 (8.3736, 8.81) -> (8.4968, 8.6869)
  arc A205 (8.3736, 9.0564) -> (8.3736, 8.81) centre (8.4968, 8.9332) ccw
  line L213 (8.8838, 9.5665) -> (8.3736, 9.0564)
  line L214 (8.3535, 10.0967) -> (8.8838, 9.5665)
  line L215 (7.8434, 9.5866) -> (8.3535, 10.0967)
  arc A206 (7.5971, 9.5866) -> (7.8434, 9.5866) centre (7.7202, 9.7098) ccw
  line L216 (7.4739, 9.7098) -> (7.5971, 9.5866)
  arc A207 (7.4739, 9.9561) -> (7.4739, 9.7098) centre (7.5971, 9.8329) ccw
  line L217 (7.9841, 10.4662) -> (7.4739, 9.9561)
  line L218 (7.4538, 10.9965) -> (7.9841, 10.4662)
  line L219 (6.9437, 10.4863) -> (7.4538, 10.9965)
  arc A208 (6.6973, 10.4863) -> (6.9437, 10.4863) centre (6.8205, 10.6095) ccw
  line L220 (6.5742, 10.6095) -> (6.6973, 10.4863)
  arc A209 (6.5742, 10.8558) -> (6.5742, 10.6095) centre (6.6973, 10.7327) ccw
  line L221 (7.0843, 11.366) -> (6.5742, 10.8558)
  line L222 (6.7526, 11.6976) -> (7.0843, 11.366)
  line L223 (8.8721, 13.8171) -> (6.7526, 11.6976)
  line L224 (9.6792, -2.5692) -> (11.6225, -0.6259)
  arc A210 (9.5661, -2.5692) -> (9.6792, -2.5692) centre (9.6227, -2.5126) ccw
  line L225 (8.5435, -1.5466) -> (9.5661, -2.5692)
  arc A211 (8.5435, -1.4334) -> (8.5435, -1.5466) centre (8.6, -1.49) ccw
  line L226 (10.4868, 0.5099) -> (8.5435, -1.4334)
  arc A212 (10.5999, 0.5099) -> (10.4868, 0.5099) centre (10.5433, 0.4533) ccw
  line L227 (11.6225, -0.5128) -> (10.5999, 0.5099)
  arc A213 (11.6225, -0.6259) -> (11.6225, -0.5128) centre (11.566, -0.5693) ccw
  line L228 (0.5538, 8.0568) -> (1.2737, 8.7766)
  arc A214 (0.4407, 8.0568) -> (0.5538, 8.0568) centre (0.4973, 8.1133) ccw
  line L229 (-1.3959, 9.8933) -> (0.4407, 8.0568)
  arc A215 (-1.3959, 10.0065) -> (-1.3959, 9.8933) centre (-1.3393, 9.9499) ccw
  line L230 (-0.6761, 10.7263) -> (-1.3959, 10.0065)
  arc A216 (-0.5629, 10.7263) -> (-0.6761, 10.7263) centre (-0.6195, 10.6697) ccw
  line L231 (1.2737, 8.8897) -> (-0.5629, 10.7263)
  arc A217 (1.2737, 8.7766) -> (1.2737, 8.8897) centre (1.2171, 8.8331) ccw
  line L232 (-11.4335, -0.5331) -> (-10.3432, 0.5572)
  arc A218 (-11.5466, -0.5331) -> (-11.4335, -0.5331) centre (-11.49, -0.4765) ccw
  line L233 (-12.2254, 0.1457) -> (-11.5466, -0.5331)
  arc A219 (-12.2254, 0.2588) -> (-12.2254, 0.1457) centre (-12.1688, 0.2023) ccw
  line L234 (-11.1351, 1.3491) -> (-12.2254, 0.2588)
  arc A220 (-11.022, 1.3491) -> (-11.1351, 1.3491) centre (-11.0786, 1.2925) ccw
  line L235 (-10.3432, 0.6703) -> (-11.022, 1.3491)
  arc A221 (-10.3432, 0.5572) -> (-10.3432, 0.6703) centre (-10.3998, 0.6137) ccw
  line L236 (-12.836, 0.7898) -> (-11.7059, 1.9198)
  arc A222 (-12.9491, 0.7898) -> (-12.836, 0.7898) centre (-12.8925, 0.8463) ccw
  line L237 (-13.6589, 1.4995) -> (-12.9491, 0.7898)
  arc A223 (-13.6589, 1.6127) -> (-13.6589, 1.4995) centre (-13.6023, 1.5561) ccw
  line L238 (-12.5288, 2.7428) -> (-13.6589, 1.6127)
  arc A224 (-12.4157, 2.7428) -> (-12.5288, 2.7428) centre (-12.4722, 2.6862) ccw
  line L239 (-11.7059, 2.033) -> (-12.4157, 2.7428)
  arc A225 (-11.7059, 1.9198) -> (-11.7059, 2.033) centre (-11.7624, 1.9764) ccw
  line L240 (-5.5283, 1.6867) -> (-2.8273, 4.3878)
  arc A226 (-5.6415, 1.6867) -> (-5.5283, 1.6867) centre (-5.5849, 1.7433) ccw
  line L241 (-8.3509, 4.3961) -> (-5.6415, 1.6867)
  arc A227 (-8.3509, 4.5092) -> (-8.3509, 4.3961) centre (-8.2943, 4.4527) ccw
  line L242 (-5.6498, 7.2103) -> (-8.3509, 4.5092)
  arc A228 (-5.5367, 7.2103) -> (-5.6498, 7.2103) centre (-5.5932, 7.1537) ccw
  line L243 (-2.8273, 4.5009) -> (-5.5367, 7.2103)
  arc A229 (-2.8273, 4.3878) -> (-2.8273, 4.5009) centre (-2.8838, 4.4443) ccw
  circle A230 centre (14.3189, -9.0863) radius 0.75
  circle A231 centre (12.5158, -10.8894) radius 0.75
  circle A232 centre (10.7127, -12.6926) radius 0.75
  circle A233 centre (8.9095, -14.4957) radius 0.75
  circle A234 centre (7.1064, -16.2988) radius 0.75
  circle A235 centre (5.3033, -18.1019) radius 0.75
  circle A236 centre (-6.9862, 12.5016) radius 0.75
  circle A237 centre (6.0104, 17.3948) radius 0.75
  circle A238 centre (16.7938, 6.47) radius 0.75
  circle A239 centre (16.6524, 2.7224) radius 0.75
  circle A240 centre (13.6118, 1.8738) radius 0.75
  circle A241 centre (11.8087, 3.677) radius 0.75
  circle A242 centre (-12.5158, 10.8187) radius 0.75
  circle A243 centre (-14.3189, 9.0156) radius 0.75
  circle A244 centre (-16.122, 7.2125) radius 0.75
  circle A245 centre (-8.7893, 10.6985) radius 0.75
  circle A246 centre (-10.5925, 8.8954) radius 0.75
  circle A247 centre (-12.3956, 7.0923) radius 0.75
  circle A248 centre (-10.7127, 12.6219) radius 0.75
  circle A249 centre (-8.9095, 14.425) radius 0.75
  circle A250 centre (-14.1987, 5.2892) radius 0.75
  circle A251 centre (-7.2478, -8.8742) radius 0.6
  circle A252 centre (-6.1872, -9.9349) radius 0.6
  circle A253 centre (-5.1265, -10.9955) radius 0.6
  circle A254 centre (-0.1768, -15.521) radius 0.6
  circle A255 centre (1.9445, -17.6423) radius 0.6
  circle A256 centre (0.8485, -16.5463) radius 0.65
  circle A257 centre (-8.9377, 0.7782) radius 0.5
  circle A258 centre (-8.8564, -0.5181) radius 0.5
  circle A259 centre (21.5668, 0) radius 2.725
  circle A260 centre (0, -21.5668) radius 2.725
  circle A261 centre (-21.5668, 0) radius 2.725
  circle A262 centre (0, 21.5668) radius 2.725
  circle A263 centre (21.5668, 0) radius 1.75
  circle A264 centre (0, -21.5668) radius 1.75
  circle A265 centre (-21.5668, 0) radius 1.75
  circle A266 centre (0, 21.5668) radius 1.75
  point P0 (0, 0)
  point P1 (0, 0)
  point P2 (2.725, 21.5668)
  point P3 (-2.3228, 22.9916)
  point P4 (22.9916, -2.3228)
  point P5 (23.2155, 2.1696)
  point P6 (-22.9916, 2.3228)
  point P7 (-2.6701, -21.0224)
  point P8 (2.3228, -22.9916)
  dimension "d19" = 2.725
  dimension "d20" = 3.5
  dimension "d21" = 3.5
  dimension "d22" = 3.5
  dimension "d23" = 3.5
  constraints: 488 end point, 444 point on circle, 267 centre point, 8 coincident, 3 concentric
  measures "d19" radius of A0
  measures "d20" diameter of A263
  measures "d21" diameter of A264
  measures "d22" diameter of A265
  measures "d23" diameter of A266
extrude "Extrusion6" cut sketch "Sketch4" against normal blind 25.4 contours A263 | A264 | A265 | A266
body "Solid2"
